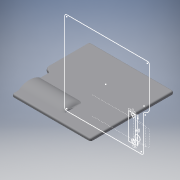
# Autodesk Inventor part: 02_Beamer_Deckel
Saved by Autodesk Inventor 2016 (Build 200138000, 138)
## iProperties
Created: 2016-09-10
Part Number: 02_Beamer_Deckel
Material: Generisch
Document SubType Name: Modeling
Designer: Bene
Density: 1 g/cm^3
Appearance: Vorgabe
Mass: 65.3023 g
Surface Area: 330.586 cm^2
Volume: 65.3023 cm^3
Author: Bene
Autodesk Inventor part; units mm, degrees
ref_plane "YZ Plane" through (0, 0, 0) normal (1, 0, 0) x (0, 1, 0)
ref_plane "XZ Plane" through (0, 0, 0) normal (0, 1, 0) x (-1, 0, 0)
ref_plane "XY Plane" through (0, 0, 0) normal (0, 0, 1) x (1, 0, 0)
sketch "Skizze1" plane through (0, 0, 0) normal (0, 0, 1) x (1, 0, 0)
  line L0 (-55, -26.5627) -> (-53, -26.5627) projected
  line L1 (-53, -26.5627) -> (-53, -8.8167) projected
  arc A0 (-53, -8.8167) -> (-57.0909, -3.9) centre (-58, -8.8167) ccw projected
  arc A1 (-62, 2) -> (-57.0909, -3.9) centre (-56, 2) ccw projected
  line L2 (-62, 2) -> (-62, 60) projected
  arc A2 (-61, 61) -> (-62, 60) centre (-61, 60) ccw projected
  line L3 (-61, 61) -> (61, 61) projected
  arc A3 (62, 60) -> (61, 61) centre (61, 60) ccw projected
  line L4 (62, 60) -> (62, -60) projected
  arc A4 (61, -61) -> (62, -60) centre (61, -60) ccw projected
  line L5 (61, -61) -> (-52, -61) projected
  arc A5 (-53, -60) -> (-52, -61) centre (-52, -60) ccw projected
  line L6 (-53, -60) -> (-53, -46.4373) projected
  line L7 (-53, -46.4373) -> (-55, -46.4373) projected
  line L8 (-55, -46.4373) -> (-55, -60) projected
  arc A6 (-55, -60) -> (-52, -63) centre (-52, -60) ccw projected
  line L9 (-52, -63) -> (61, -63) projected
  arc A7 (61, -63) -> (64, -60) centre (61, -60) ccw projected
  line L10 (64, -60) -> (64, 60) projected
  arc A8 (64, 60) -> (61, 63) centre (61, 60) ccw projected
  line L11 (61, 63) -> (-61, 63) projected
  arc A9 (-61, 63) -> (-64, 60) centre (-61, 60) ccw projected
  line L12 (-64, 60) -> (-64, 2) projected
  arc A10 (-64, 2) -> (-57.4545, -5.8667) centre (-56, 2) ccw projected
  arc A11 (-55, -8.8167) -> (-57.4545, -5.8667) centre (-58, -8.8167) ccw projected
  line L13 (-55, -8.8167) -> (-55, -26.5627) projected
  line L14 (-53, -15.5) -> (-53, -28.7058) projected
  line L15 (-55, -57.5) -> (-55, -15.5) projected
  point P0 (0, 0)
extrude "Extrusion1" add sketch "Skizze1" along normal blind 4
sketch "Skizze2" plane through (-55, -60, 0) normal (-1, 0, 0) x (0, 0, 1)
  arc A0 (0, 33.4373) -> (0, 13.5627) centre (-18.5, 23.5) ccw projected
  circle A1 centre (-18.5, 23.5) radius 21
  point P0 (0, 60)
  constraints: 1 centre point, 1 coincident, 1 concentric
extrude "Extrusion2" cut sketch "Skizze2" against normal blind 68
fillet "Rundung2" radius 2 11 edges at (4.5, -63, 4) (63.1213, -62.1213, 4) (64, 0, 4) (63.1213, 62.1213, 4) (0, 63, 4) (-63.1213, 62.1213, 4) (-64, 31, 4) (-62.1496, -3.1168, 4) (-55.6939, -6.8978, 4) (-55, -34.4083, 4) (-54.1213, -62.1213, 4)
